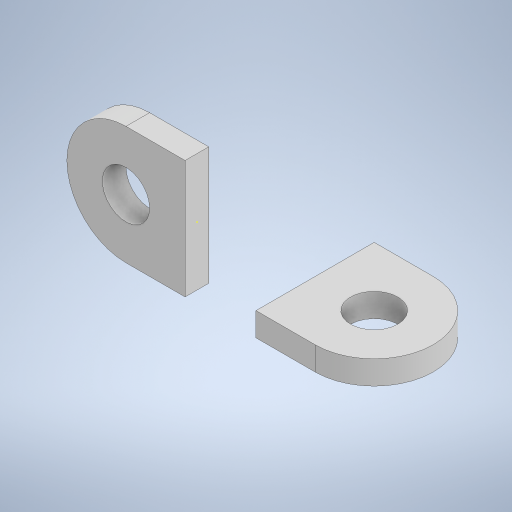
# Autodesk Inventor part: loft
Saved by Autodesk Inventor 2023 (Build 270158000, 158)
## iProperties
Created: 2023-07-03
Part Number: loft
Material: Generico
Document SubType Name: Modeling
Designer: nicol
Density: 1 g/cm^3
Appearance: Default
Author: nicol
Autodesk Inventor part; units mm, degrees
ref_plane "YZ Plane" through (0, 0, 0) normal (1, 0, 0) x (0, 1, 0)
ref_plane "XZ Plane" through (0, 0, 0) normal (0, 1, 0) x (-1, 0, 0)
ref_plane "XY Plane" through (0, 0, 0) normal (0, 0, 1) x (1, 0, 0)
sketch "Schizzo1" plane through (0, 0, 0) normal (1, 0, 0) x (0, 1, 0)
  line L0 (25, 5) -> (-25, 5)
  line L1 (-25, 5) -> (-25, -5)
  line L2 (-25, -5) -> (25, -5)
  line L3 (25, -5) -> (25, 5)
  line L4 (25, 5) -> (-25, -5) construction
  line L5 (-25, 5) -> (25, -5) construction
  point P0 (0, 0)
  dimension "d0" = 50
  dimension "d1" = 10
  constraints: 12 end point, 2 midpoint, 2 parallel, 1 horizontal, 1 perpendicular
  measures "d0" distance of L2.end L1.end
  measures "d1" distance of L1.end L0.end
extrude "Estrusione1" add sketch "Schizzo1" along normal blind 50
ref_plane "Piano di lavoro1" through (100, 0, 0) normal (1, 0, 0) x (0, 0, -1)
sketch "Schizzo2" plane through (50, 0, 0) normal (1, 0, 0) x (0, 0, -1)
  point P0 (0, 0)
sketch "Schizzo3" plane through (100, 0, 0) normal (1, 0, 0) x (0, 0, -1)
  line L0 (-25, 5) -> (25, 5)
  line L1 (25, 5) -> (25, -5)
  line L2 (25, -5) -> (-25, -5)
  line L3 (-25, -5) -> (-25, 5)
  line L4 (-25, 5) -> (25, -5) construction
  line L5 (25, 5) -> (-25, -5) construction
  point P0 (0, 0)
  dimension "d5" = 50
  dimension "d6" = 10
  constraints: 12 end point, 2 midpoint, 2 parallel, 1 horizontal, 1 perpendicular
  measures "d5" distance of L1.end L2.end
  measures "d6" distance of L0.end L1.end
extrude "Estrusione2" add sketch "Schizzo3" along normal blind 50
fillet "Raccordo1" radius 25 4 edges at (150, 0, 25) (150, 0, -25) (0, 25, 0) (0, -25, 0)
sketch "Schizzo4" plane through (50, -25, 5) normal (0, 0, 1) x (1, 0, 0)
  arc A0 (-25, 50) -> (-25, 0) centre (-25, 25) ccw projected
  point P0 (-50, 25)
  constraints: 1 coincident
hole "Foro1" at (25, 0, 5) direction (0, 0, -1) diameter 20 end through all
sketch "Schizzo5" plane through (100, 5, 25) normal (0, 1, 0) x (1, 0, 0)
  arc A0 (25, 0) -> (25, 50) centre (25, 25) ccw projected
  point P0 (-100, 25)
  constraints: 1 coincident
hole "Foro2" at (125, 5, 0) direction (0, -1, 0) diameter 20 end through all
